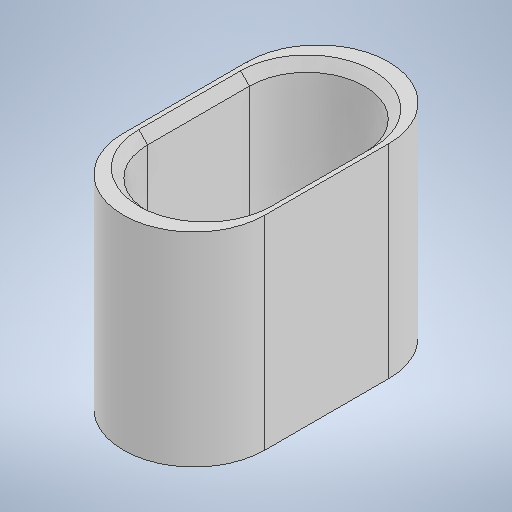
# Autodesk Inventor part: motor-tuningpeg
Saved by Autodesk Inventor 2025.2 (Build 292293000, 293)
## iProperties
Created: 2025-03-05
Part Number: motor-tuningpeg
Material: Generic
Document SubType Name: Modeling
Designer: 3lin2
Density: 1 g/cm^3
Appearance: Default
Author: 3lin2
Autodesk Inventor part; units mm, degrees
ref_plane "YZ Plane" through (0, 0, 0) normal (1, 0, 0) x (0, 1, 0)
ref_plane "XZ Plane" through (0, 0, 0) normal (0, 1, 0) x (-1, 0, 0)
ref_plane "XY Plane" through (0, 0, 0) normal (0, 0, 1) x (1, 0, 0)
sketch "Sketch1" plane through (0, 0, 0) normal (0, 1, 0) x (-1, 0, 0)
  line L0 (-0.0001, 4.0208) -> (-0.0001, -8.9792) construction
  line L1 (0, 7) -> (0, -7) construction
  line L2 (-8, 7) -> (-8, -7)
  line L3 (8, -7) -> (8, 7)
  arc A0 (8, 7) -> (-8, 7) centre (0, 7) ccw
  arc A1 (-8, -7) -> (8, -7) centre (0, -7) ccw
  point P0 (0, 0)
  point P1 (0, 0)
  point P2 (0, -15)
  point P3 (0, 15)
  dimension "d4" = 16
  dimension "d5" = 30
  constraints: 12 end point, 6 point on circle, 4 tangent, 2 centre point, 2 vertical, 1 coincident, 1 midpoint, 1 parallel
  measures "d4" diameter of A1
  measures "d5" distance of point (0, -15) point (0, 15)
extrude "Extrusion1" add sketch "Sketch1" along normal blind 23
sketch "Sketch4" plane through (0, 23, 0) normal (0, 1, 0) x (1, 0, 0)
  line L0 (0.0016, 5.7534) -> (0.0016, -5.7466) construction
  line L1 (-6.4984, 5.7534) -> (-6.4984, -5.7466)
  line L2 (6.5016, -5.7466) -> (6.5016, 5.7534)
  arc A0 (6.5016, 5.7534) -> (-6.4984, 5.7534) centre (0.0016, 5.7534) ccw
  arc A1 (-6.4984, -5.7466) -> (6.5016, -5.7466) centre (0.0016, -5.7466) ccw
  point P0 (0, 0)
  point P1 (0.0016, 0.0034)
  point P2 (0.0016, -12.2466)
  point P3 (0.0016, 12.2534)
  point P4 (6.5016, 0.0034)
  point P5 (-6.4984, 0.0034)
  dimension "d11" = 24.5
  dimension "d12" = 13
  constraints: 8 end point, 6 point on circle, 4 tangent, 3 midpoint, 2 centre point, 1 parallel, 1 vertical
  measures "d11" distance of point (0.002, -12.247) point (0.002, 12.253)
  measures "d12" distance of point (6.502, 0.003) point (-6.498, 0.003)
extrude "Extrusion2" cut sketch "Sketch4" against normal blind 18
sketch "Sketch5" plane through (0, 0, 0) normal (0, -1, 0) x (1, 0, 0)
  circle A0 centre (0, 0) radius 1.9
  line L0 (1.3856, -1.3) -> (-1.3856, -1.3)
  point P0 (0, -1.3)
  dimension "d15" = 3.8
  dimension "d16" = 1.3
  constraints: 2 end point, 2 point on circle, 1 centre point, 1 coincident, 1 horizontal, 1 midpoint
  measures "d15" diameter of A0
  measures "d16" distance of A0.centre point (0, -1.3)
extrude "Extrusion3" cut sketch "Sketch5" against normal blind 18 contours A0 L0 picked at (0.0696, -0.2372)
chamfer "Chamfer1" distance 1 angle 45 4 edges at (-6.4984, 23, -0.0034) (0.0016, 23, -12.2534) (6.5016, 23, -0.0034) (0.0016, 23, 12.2466)
body "Solid1"
